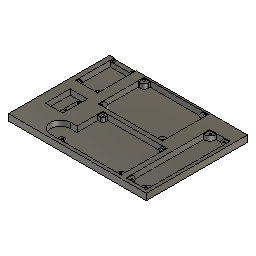
testBracket (Autodesk Fusion 360 design; units mm, degrees)
Autodesk Fusion 360 part; units mm, degrees
sketch "Sketch1" plane through (0, 0, 0) normal (0, 0, 1) x (1, 0, 0)
  line L0 (-75, 55) -> (75, 55)
  line L1 (75, 55) -> (75, -55)
  line L2 (75, -55) -> (-75, -55)
  line L3 (-75, -55) -> (-75, 55)
  line L4 (75, -55) -> (-75, 55) construction
  dimension "d1" = 150
  dimension "d2" = 110
  constraint horizontal L0
  constraint vertical L1
  constraint horizontal L2
  constraint vertical L3
  constraint midpoint origin L4
  measures "d1" distance of L0.start L0.end
  measures "d2" distance of L0.start L2.end
extrude "Extrude1" add sketch "Sketch1" along normal blind 1
sketch "Sketch2" plane through (0, 0, 1) normal (0, 0, 1) x (-1, 0, 0)
  line L0 (75, 55) -> (-75, 55)
  line L1 (-75, 55) -> (-75, -55)
  line L2 (-75, -55) -> (75, -55)
  line L3 (75, -55) -> (75, 55)
  line L4 (35.5, -53) -> (-34.5, -53)
  line L5 (-34.5, -53) -> (-34.5, -3)
  line L6 (-34.5, -3) -> (35.5, -3)
  line L7 (35.5, -3) -> (35.5, -53)
  line L8 (26, 1.5) -> (-44, 1.5)
  line L9 (-44, 1.5) -> (-44, 51.5)
  line L10 (-44, 51.5) -> (26, 51.5)
  line L11 (26, 51.5) -> (26, 1.5)
  line L12 (-49.5, -39.5) -> (-71.5, -39.5)
  line L13 (-71.5, -39.5) -> (-71.5, 51.5)
  line L14 (-71.5, 51.5) -> (-49.5, 51.5)
  line L15 (-49.5, 51.5) -> (-49.5, -39.5)
  line L16 (65, -2) -> (46, -2)
  line L17 (46, -2) -> (46, 25)
  line L18 (46, 25) -> (65, 25)
  line L19 (65, 25) -> (65, -2)
  arc A0 (33, 29.5) -> (33, 51.5) centre (33, 40.5) ccw
  line L20 (33, 29.5) -> (26, 29.5)
  line L21 (33, 51.5) -> (26, 51.5)
  line L22 (70, -55) -> (46, -55)
  line L23 (46, -55) -> (46, -13)
  line L24 (46, -13) -> (70, -13)
  line L25 (70, -13) -> (70, -55)
  point P0 (26, 40.5)
  point P1 (33, 40.5)
  dimension "d5" = 70
  dimension "d6" = 50
  dimension "d7" = 70
  dimension "d8" = 50
  dimension "d9" = 22
  dimension "d10" = 91
  dimension "d11" = 19
  dimension "d12" = 27
  dimension "d13" = 3.5
  dimension "d14" = 3.5
  dimension "d15" = 3.5
  dimension "d16" = 2
  dimension "d18" = 10
  dimension "d20" = 20
  dimension "d21" = 5.5
  dimension "d22" = 30
  dimension "d23" = 15
  dimension "d37" = 11
  dimension "d38" = 7
  dimension "d39" = 11
  dimension "d47" = 24
  dimension "d48" = 42
  dimension "d49" = 5
  constraint horizontal L4
  constraint vertical L5
  constraint horizontal L6
  constraint vertical L7
  constraint horizontal L8
  constraint vertical L9
  constraint horizontal L10
  constraint vertical L11
  constraint horizontal L12
  constraint vertical L13
  constraint horizontal L14
  constraint vertical L15
  constraint horizontal L16
  constraint vertical L17
  constraint horizontal L18
  constraint vertical L19
  constraint coincident L11 P0
  constraint coincident P1 A0.centre
  constraint coincident L11 L20.end
  constraint tangent A0 L20
  constraint perpendicular L11 L20
  constraint tangent A0 L21
  constraint horizontal L22
  constraint vertical L23
  constraint horizontal L24
  constraint vertical L25
  constraint coincident L2 L22.start
  measures "d5" distance of L4.start L4.end
  measures "d6" distance of L4.start L6.end
  measures "d7" distance of L8.start L8.end
  measures "d8" distance of L8.start L10.end
  measures "d9" distance of L12.start L12.end
  measures "d10" distance of L12.start L14.end
  measures "d11" distance of L16.start L16.end
  measures "d12" distance of L16.start L18.end
  measures "d13" distance of L1 L13
  measures "d14" distance of L0 L14
  measures "d15" distance of L0 L10
  measures "d16" distance of L2 L4
  measures "d18" distance of L3 L19
  measures "d20" distance of L11 L17
  measures "d21" distance of L9 L15
  measures "d22" distance of L0 L18
  measures "d23" distance of L5 L15
  measures "d37" distance of L10.end P0
  measures "d38" distance of P0 P1
  measures "d39" radius of A0
  measures "d47" distance of L22.start L22.end
  measures "d48" distance of L22.start L24.end
  measures "d49" distance of L3 L25
extrude "Extrude2" add sketch "Sketch2" along normal blind 6 contours L0 L1 L2 L3 L23 L24 L25
sketch "Sketch3" plane through (0, 0, 1) normal (0, 0, 1) x (-1, 0, 0)
  line L0 (-71.5, -39.5) -> (-71.5, 51.5)
  line L1 (-71.5, 51.5) -> (-49.5, 51.5)
  line L2 (-49.5, 51.5) -> (-49.5, -39.5)
  line L3 (-49.5, -39.5) -> (-71.5, -39.5)
  circle A0 centre (-53, -36.5) radius 1
  line L4 (-68, 48.5) -> (-53, -36.5) construction
  line L5 (-71.5, -39.5) -> (-49.5, 51.5) construction
  circle A1 centre (-68, -36.5) radius 1
  circle A2 centre (-53, 48.5) radius 1
  circle A3 centre (-68, 48.5) radius 1
  arc A4 (-64.5, -39.5) -> (-71.5, -32.5) centre (-71.5, -39.5) ccw
  arc A5 (-49.5, -32.5) -> (-56.5, -39.5) centre (-49.5, -39.5) ccw
  arc A6 (-71.5, 44.5) -> (-64.5, 51.5) centre (-71.5, 51.5) ccw
  arc A7 (-56.5, 51.5) -> (-49.5, 44.5) centre (-49.5, 51.5) ccw
  dimension "d24" = 2
  dimension "d27" = -15
  dimension "d28" = 85
  dimension "d29" = 7
  dimension "d30" = 7
  dimension "d31" = 7
  dimension "d32" = 7
  constraint coincident L4.start A3.centre
  constraint coincident A0.centre L4.end
  constraint coincident L0.start L3.end
  constraint coincident L1.end L2.start
  constraint midpoint L4 L5
  constraint coincident L0 A4.end
  constraint coincident L3 A4.start
  constraint coincident L2 A5.start
  constraint coincident L2.end L3.start
  constraint coincident L1 A6.end
  constraint coincident L0.end L1.start
  constraint coincident L2 A7.end
  constraint coincident L1 A7.start
  measures "d24" diameter of A0
  measures "d29" radius of A4
  measures "d30" radius of A5
  measures "d31" radius of A6
  measures "d32" radius of A7
sketch "Sketch4" plane through (0, 0, 1) normal (0, 0, 1) x (-1, 0, 0)
  line L0 (46, 25) -> (46, -2)
  line L1 (46, -2) -> (65, -2)
  line L2 (65, -2) -> (65, 25)
  line L3 (65, 25) -> (46, 25)
  circle A0 centre (48, 5.9) radius 1
  circle A1 centre (48, 19.4) radius 1
  line L4 (46, -2) -> (46, 25)
  line L5 (46, 25) -> (65, 25)
  arc A2 (48, 3.4) -> (50.5, 5.9) centre (48, 5.9) ccw
  line L6 (48, 3.4) -> (46, 3.4)
  line L7 (50.5, 5.9) -> (50.5, 25)
  dimension "d40" = 2
  dimension "d41" = 2
  dimension "d42" = 13.5
  dimension "d43" = 2
  dimension "d44" = 5.6
  dimension "d45" = 7.9
  dimension "d46" = 2.5
  constraint coincident A0.centre A2.centre
  constraint coincident L4 L6.end
  constraint tangent A2 L6
  constraint perpendicular L4 L6
  constraint coincident L5 L7.end
  constraint tangent A2 L7
  constraint perpendicular L5 L7
  measures "d40" diameter of A0
  measures "d41" diameter of A1
  measures "d42" distance of A0.centre A1.centre
  measures "d43" distance of A0.centre L4
  measures "d44" distance of A1.centre L5
  measures "d45" distance of L1 A0.centre
  measures "d46" radius of A2
sketch "Sketch5" plane through (0, 0, 1) normal (0, 0, 1) x (-1, 0, 0)
  circle A0 centre (67.7, -52.75) radius 1
  circle A1 centre (48.3, -52.75) radius 1
  circle A2 centre (67.7, -15.25) radius 1
  circle A3 centre (48.3, -15.25) radius 1
  line L0 (67.7, -52.75) -> (48.3, -15.25) construction
  line L1 (46, -13) -> (46, -55) construction
  line L2 (46, -55) -> (70, -55) construction
  line L3 (70, -55) -> (70, -13) construction
  line L4 (70, -13) -> (46, -13) construction
  line L5 (46, -55) -> (70, -13) construction
  line L6 (70, -50.5) -> (46, -50.5)
  line L7 (70, -55) -> (46, -55)
  arc A4 (48.3, -17.25) -> (50.3, -15.25) centre (48.3, -15.25) ccw
  arc A5 (65.7, -15.25) -> (67.7, -17.25) centre (67.7, -15.25) ccw
  line L8 (67.7, -17.25) -> (70, -17.25)
  line L9 (65.7, -15.25) -> (65.7, -13)
  line L10 (50.3, -15.25) -> (50.3, -13)
  line L11 (48.3, -17.25) -> (46, -17.25)
  line L12 (70, -55) -> (70, -50.5)
  line L13 (46, -50.5) -> (46, -55)
  line L14 (50.3, -13) -> (46, -13)
  line L15 (46, -17.25) -> (46, -13)
  line L16 (70, -17.25) -> (70, -13)
  line L17 (70, -13) -> (65.7, -13)
  dimension "d50" = 2
  dimension "d53" = -19.4
  dimension "d54" = 37.5
  dimension "d55" = 2.25
  dimension "d56" = 2.25
  dimension "d57" = 2
  dimension "d58" = 2
  constraint coincident A0.centre L0.start
  constraint coincident A3.centre L0.end
  constraint coincident L1.end L2.start
  constraint coincident L3.end L4.start
  constraint midpoint L0 L5
  constraint coincident L3 L6.start
  constraint coincident L1 L6.end
  constraint perpendicular L1 L6
  constraint coincident A2.centre A5.centre
  constraint coincident L3 L8.end
  constraint tangent A5 L8
  constraint perpendicular L3 L8
  constraint coincident L4 L9.end
  constraint tangent A5 L9
  constraint perpendicular L4 L9
  constraint coincident L4 L10.end
  constraint tangent A4 L10
  constraint perpendicular L4 L10
  constraint coincident L1 L11.end
  constraint tangent A4 L11
  constraint perpendicular L1 L11
  constraint coincident L2.end L3.start
  constraint coincident L1.start L4.end
  measures "d50" diameter of A0
  measures "d55" distance of A1.centre L7
  measures "d56" distance of A1.centre L6
  measures "d57" radius of A4
  measures "d58" radius of A5
sketch "Sketch6" plane through (0, 0, 1) normal (0, 0, 1) x (1, 0, 0)
  line L0 (-35.5, 53) -> (34.5, 53)
  line L1 (-35.5, 3) -> (-35.5, 53)
  line L2 (34.5, 53) -> (34.5, 3)
  line L3 (34.5, 3) -> (-35.5, 3)
  circle A0 centre (-33.5, 5) radius 1
  line L4 (-33.5, 51) -> (32.5, 5) construction
  line L5 (34.5, 53) -> (-35.5, 3) construction
  circle A1 centre (32.5, 5) radius 1
  circle A2 centre (-33.5, 51) radius 1
  circle A3 centre (32.5, 51) radius 1
  arc A4 (-33.5, 46.5) -> (-29, 51) centre (-33.5, 51) ccw
  line L6 (-29, 51) -> (-29, 53)
  line L7 (-33.5, 46.5) -> (-35.5, 46.5)
  line L8 (28, 5) -> (28, 3)
  arc A5 (32.5, 9.5) -> (28, 5) centre (32.5, 5) ccw
  line L9 (32.5, 9.5) -> (34.5, 9.5)
  arc A6 (28, 51) -> (32.5, 46.5) centre (32.5, 51) ccw
  line L10 (32.5, 46.5) -> (34.5, 46.5)
  line L11 (28, 51) -> (28, 53)
  arc A7 (-29, 5) -> (-33.5, 9.5) centre (-33.5, 5) ccw
  line L12 (-33.5, 9.5) -> (-35.5, 9.5)
  line L13 (-29, 5) -> (-29, 3)
  point P0 (-0.5, 28)
  dimension "d59" = 2
  dimension "d62" = 66
  dimension "d63" = 46
  dimension "d64" = 4.5
  dimension "d66" = 360
  dimension "d67" = 4.5
  constraint coincident L4.start A2.centre
  constraint coincident L4.end A1.centre
  constraint coincident L0.end L2.start
  constraint coincident L1.start L3.end
  constraint midpoint L4 L5
  constraint coincident L0 L6.end
  constraint tangent A4 L6
  constraint perpendicular L0 L6
  constraint coincident L1 L7.end
  constraint tangent A4 L7
  constraint perpendicular L1 L7
  constraint midpoint L5 P0
  constraint coincident A3.centre A6.centre
  constraint coincident L2 L10.end
  constraint tangent A6 L10
  constraint perpendicular L2 L10
  constraint coincident L0 L11.end
  constraint tangent A6 L11
  constraint perpendicular L0 L11
  measures "d59" diameter of A0
  measures "d64" radius of A4
  measures "d67" radius of A6
sketch "Sketch7" plane through (0, 0, 1) normal (0, 0, 1) x (-1, 0, 0)
  arc A0 (33, 29.5) -> (33, 51.5) centre (33, 40.5) ccw
  circle A1 centre (-41, 4.25) radius 1
  circle A2 centre (23, 4.25) radius 1
  circle A3 centre (-41, 48.75) radius 1
  circle A4 centre (23, 48.75) radius 1
  line L0 (26, 29.5) -> (26, 1.5) construction
  line L1 (26, 1.5) -> (-44, 1.5) construction
  line L2 (-44, 1.5) -> (-44, 51.5) construction
  line L3 (-44, 51.5) -> (33, 51.5) construction
  line L4 (33, 29.5) -> (26, 29.5) construction
  arc A5 (33, 29.5) -> (33, 51.5) centre (33, 40.5) ccw construction
  line L5 (26, 1.5) -> (-44, 51.5) construction
  line L6 (-41, 4.25) -> (23, 48.75) construction
  arc A6 (23, 6.75) -> (20.5, 4.25) centre (23, 4.25) ccw
  line L7 (20.5, 4.25) -> (20.5, 1.5)
  line L8 (23, 6.75) -> (26, 6.75)
  line L9 (26, 6.75) -> (26, 1.5)
  line L10 (26, 1.5) -> (20.5, 1.5)
  line L11 (-44, 51.5) -> (-38.5, 51.5)
  line L12 (-44, 46.25) -> (-44, 51.5)
  circle A7 centre (-41, 48.75) radius 1
  line L13 (-38.5, 48.75) -> (-38.5, 51.5)
  arc A8 (-41, 46.25) -> (-38.5, 48.75) centre (-41, 48.75) ccw
  line L14 (-41, 46.25) -> (-44, 46.25)
  arc A9 (-38.5, 4.25) -> (-41, 6.75) centre (-41, 4.25) ccw
  line L15 (-41, 4.25) -> (-38.5, 4.25) construction
  line L16 (-41, 4.25) -> (-41, 6.75) construction
  line L17 (-41, 6.75) -> (-44, 6.75)
  line L18 (-38.5, 4.25) -> (-38.5, 1.5)
  line L19 (-38.5, 1.5) -> (-44, 1.5)
  line L20 (-44, 1.5) -> (-44, 6.75)
  line L21 (26, 51.5) -> (26, 46.25)
  line L22 (20.5, 51.5) -> (26, 51.5)
  arc A10 (20.5, 48.75) -> (23, 46.25) centre (23, 48.75) ccw
  line L23 (23, 46.25) -> (26, 46.25)
  line L24 (20.5, 48.75) -> (20.5, 51.5)
  circle A11 centre (23, 48.75) radius 1
  point P0 (-9, 26.5)
  dimension "d77" = 2
  dimension "d80" = 64
  dimension "d81" = 44.5
  dimension "d82" = 2.5
  dimension "d84" = 360
  dimension "d85" = 2.5
  dimension "d86" = 90
  constraint coincident L0.end L1.start
  constraint coincident L2.end L3.start
  constraint coincident A1.centre L6.start
  constraint coincident A4.centre L6.end
  constraint midpoint L5 L6
  constraint coincident A2.centre A6.centre
  constraint coincident L1 L7.end
  constraint tangent A6 L7
  constraint perpendicular L1 L7
  constraint coincident L0 L8.end
  constraint tangent A6 L8
  constraint perpendicular L0 L8
  constraint midpoint L5 P0
  constraint coincident L2 L17.end
  constraint tangent A9 L17
  constraint perpendicular L2 L17
  constraint coincident L1 L18.end
  constraint tangent A9 L18
  constraint coincident L1.end L2.start
  measures "d77" diameter of A1
  measures "d82" radius of A6
  measures "d85" radius of A9
  measures "d86" angle of L15 L16
extrude "Extrude3" add sketch "Sketch5" sketch "Sketch6" sketch "Sketch3" sketch "Sketch7" sketch "Sketch4" along normal blind 5 of sketch 2 contours L0 L1 A4 L6 L7 | L0 L2 A6 L10 L11 | L1 L3 A7 L12 L13 | L2 L3 L8 A5 L9 of sketch 3 contours L0 L3 A4 | L0 L1 A6 | L2 L3 A5 | L1 L2 A7 of sketch 4 of sketch 5 contours L0 L3 L4 L5 A2 L6 L7
equation "d15 = d14"
equation "d38 = 18 mm - 11 mm"
equation "d56 = d55"
